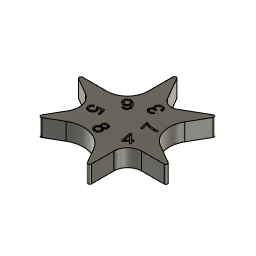
RadiusTool (Autodesk Fusion 360 design; units mm, degrees)
Autodesk Fusion 360 part; units mm, degrees
sketch "Sketch1" plane through (0, 0, 0) normal (0, 0, 1) x (1, 0, 0)
  circle A0 centre (0, 0) radius 20
  line L0 (-4.0272, 3.9759) -> (-4.0272, 20)
  line L1 (-20, 3.9759) -> (-4.0272, 3.9759)
  line L2 (20, -6) -> (6, -6)
  line L3 (6, -6) -> (6, -20)
  dimension "d1" = 40
  constraint coincident A0.centre origin
  constraint horizontal L2
  constraint vertical L3
  constraint horizontal L1
  constraint vertical L0
  measures "d1" diameter of A0
extrude "Extrude1" add sketch "Sketch1" along normal blind 5 contours A0 L0 L1 L2 L3 makes body 1
sketch "Sketch2" plane through (0, 0, 5) normal (0, 0, 1) x (-1, 0, 0)
  arc A0 (-19.0788, 6) -> (4.0272, -19.5904) centre (0, 0) ccw
  line L0 (4.0272, -19.5904) -> (4.0272, -3.9759)
  line L1 (4.0272, -3.9759) -> (19.6008, -3.9759)
  arc A1 (19.6008, -3.9759) -> (-6, 19.0788) centre (0, 0) ccw
  line L2 (-6, 19.0788) -> (-6, 6)
  line L3 (-6, 6) -> (-19.0788, 6)
copy_body "Body->Comp1" bodies 1 removing the originals makes body 2 in component "Component"
move_body "Move1" bodies 2 to x (0.5, -0.866025, 0) y (0.866025, 0.5, 0) z (0, 0, 1) at (0, 0, 0) in component "Component"
sketch "Sketch5" plane through (0, 0, 0) normal (1, 0, 0) x (0, 1, 0)
extrude "Extrude4" cut sketch "Sketch1" along normal blind 5 contours A0 L0 L1 | A0 L2 L3 sketch seen with x (0.5, 0.866025, 0) y (-0.866025, 0.5, 0) z (0, 0, 1) at (0, 0, 0) bodies 2 in component "Component"
extrude "Extrude5" cut sketch "Sketch1" along normal blind 5 contours A0 L0 L1 | A0 L2 L3 sketch seen with x (-1, 0, 0) y (0, -1, 0) z (0, 0, 1) at (0, 0, 0) bodies 2 in component "Component"
fillet "Fillet8" radius 3 1 edges at (-2.1962, -8.1962, 2.5) on bodies 2 in component "Component"
fillet "Fillet9" radius 4 1 edges at (-6, 6, 2.5) on bodies 2 in component "Component"
fillet "Fillet10" radius 5 1 edges at (8.1962, 2.1962, 2.5) on bodies 2 in component "Component"
fillet "Fillet11" radius 6 1 edges at (4.0272, -3.9759, 2.5) on bodies 2 in component "Component"
fillet "Fillet12" radius 7 1 edges at (-5.4568, -1.4997, 2.5) on bodies 2 in component "Component"
fillet "Fillet13" radius 8 1 edges at (1.4297, 5.4756, 2.5) on bodies 2 in component "Component"
fillet "Fillet14" radius 0.5 6 edges at (-6, 18.3442, 2.5) (-18.4467, 6, 2.5) (-12.8865, -14.3682, 2.5) (14.4195, 12.9753, 2.5) (18.8865, -3.9759, 2.5) (4.0272, -18.9753, 2.5) on bodies 2 in component "Component"
sketch "Sketch7" plane through (0, 0, 5) normal (0, 0, 1) x (-1, 0, 0)
  arc A0 (3.0942, -17.3593) -> (4.0272, -17.1093) centre (3.5272, -17.1093) ccw
  line L0 (4.0272, -17.1093) -> (4.0272, -9.9759)
  arc A1 (10.0272, -3.9759) -> (4.0272, -9.9759) centre (10.0272, -9.9759) ccw
  line L1 (10.0272, -3.9759) -> (17.0205, -3.9759)
  arc A2 (17.0205, -3.9759) -> (17.2705, -3.0429) centre (17.0205, -3.4759) ccw
  line L2 (17.2705, -3.0429) -> (12.5263, -0.3038)
  arc A3 (10.6962, 6.5263) -> (12.5263, -0.3038) centre (15.0263, 4.0263) ccw
  line L3 (10.6962, 6.5263) -> (13.4865, 11.3593)
  arc A4 (13.4865, 11.3593) -> (12.8035, 12.0423) centre (13.0535, 11.6093) ccw
  line L4 (12.8035, 12.0423) -> (8.3579, 9.4756)
  arc A5 (-2.5703, 12.4038) -> (8.3579, 9.4756) centre (4.3579, 16.4038) ccw
  line L5 (-2.5703, 12.4038) -> (-5.067, 16.7281)
  arc A6 (-5.067, 16.7281) -> (-6, 16.4781) centre (-5.5, 16.4781) ccw
  line L6 (-6, 16.4781) -> (-6, 10)
  arc A7 (-10, 6) -> (-6, 10) centre (-10, 10) ccw
  line L7 (-10, 6) -> (-16.5806, 6)
  arc A8 (-16.5806, 6) -> (-16.8306, 5.067) centre (-16.5806, 5.5) ccw
  line L8 (-16.8306, 5.067) -> (-11.519, 2.0003)
  arc A9 (-8.9568, -7.5619) -> (-11.519, 2.0003) centre (-15.019, -4.0619) ccw
  line L9 (-8.9568, -7.5619) -> (-11.9535, -12.7522)
  arc A10 (-11.9535, -12.7522) -> (-11.2705, -13.4352) centre (-11.5205, -13.0022) ccw
  line L10 (-11.2705, -13.4352) -> (-4.7942, -9.6962)
  arc A11 (-0.6962, -10.7942) -> (-4.7942, -9.6962) centre (-3.2942, -12.2942) ccw
  line L11 (-0.6962, -10.7942) -> (3.0942, -17.3593)
  line L12 (-3.2168, -7.9766) -> (-0.9529, -8.5832) construction
  line L13 (-0.9529, -8.5832) -> (0.3412, -3.7536) construction
  line L14 (0.3412, -3.7536) -> (-1.9227, -3.147) construction
  line L15 (-1.9227, -3.147) -> (-3.2168, -7.9766) construction
  line L16 (-5.3159, 6.9981) -> (-7.0664, 5.2476) construction
  line L17 (-7.0664, 5.2476) -> (-3.5309, 1.7121) construction
  line L18 (-3.5309, 1.7121) -> (-1.7804, 3.4626) construction
  line L19 (-1.7804, 3.4626) -> (-5.3159, 6.9981) construction
  line L20 (9.243, 1.5792) -> (8.6288, 3.8714) construction
  line L21 (8.6288, 3.8714) -> (3.7992, 2.5773) construction
  line L22 (3.7992, 2.5773) -> (4.4134, 0.2851) construction
  line L23 (4.4134, 0.2851) -> (9.243, 1.5792) construction
  line L24 (4.2315, -5.8439) -> (5.9026, -4.1728) construction
  line L25 (5.9026, -4.1728) -> (2.3671, -0.6372) construction
  line L26 (2.3671, -0.6372) -> (0.696, -2.3083) construction
  line L27 (0.696, -2.3083) -> (4.2315, -5.8439) construction
  line L28 (-7.5796, -0.5504) -> (-6.9799, -2.7884) construction
  line L29 (-6.9799, -2.7884) -> (-2.1503, -1.4943) construction
  line L30 (-2.1503, -1.4943) -> (-2.75, 0.7437) construction
  line L31 (-2.75, 0.7437) -> (-7.5796, -0.5504) construction
  line L32 (3.2162, 7.5935) -> (0.8936, 8.0031) construction
  line L33 (0.8936, 8.0031) -> (0.0254, 3.079) construction
  line L34 (0.0254, 3.079) -> (2.3479, 2.6695) construction
  line L35 (2.3479, 2.6695) -> (3.2162, 7.5935) construction
  text T0 "3" font "Arial" height 5 align ink ink in box 0 x 0 at (-3.2168, -7.9766) x (0.965926, -0.258819) y (0.258819, 0.965926) spacing 1 height is em
  text T1 "4" font "Arial" height 5 align ink ink in box 0 x 0 at (-5.3159, 6.9981) x (-0.707107, -0.707107) y (0.707107, -0.707107) spacing 1 height is em
  text T2 "5" font "Arial" height 5 align ink ink in box 0 x 0 at (9.243, 1.5792) x (-0.258819, 0.965926) y (-0.965926, -0.258819) spacing 1 height is em
  text T3 "6" font "Arial" height 5 align ink ink in box 0 x 0 at (4.2315, -5.8439) x (0.707107, 0.707107) y (-0.707107, 0.707107) spacing 1 height is em
  text T4 "7" font "Arial" height 5 align ink ink in box 0 x 0 at (-7.5796, -0.5504) x (0.258819, -0.965926) y (0.965926, 0.258819) spacing 1 height is em
  text T5 "8" font "Arial" height 5 align ink ink in box 0 x 0 at (3.2162, 7.5935) x (-0.984808, 0.173648) y (-0.173648, -0.984808) spacing 1 height is em
  constraint perpendicular L12 L13
  constraint parallel L12 L14
  constraint parallel L13 L15
  constraint perpendicular L16 L17
  constraint parallel L16 L18
  constraint parallel L17 L19
  constraint perpendicular L20 L21
  constraint parallel L20 L22
  constraint parallel L21 L23
  constraint perpendicular L24 L25
  constraint parallel L24 L26
  constraint parallel L25 L27
  constraint perpendicular L28 L29
  constraint parallel L28 L30
  constraint parallel L29 L31
  constraint perpendicular L32 L33
  constraint parallel L32 L34
  constraint parallel L33 L35
extrude "Extrude6" cut sketch "Sketch7" against normal blind 0.5 text T0 T4 T1 T5 T2 T3 sketch seen with x (-1, 0, 0) y (0, -1, 0) z (0, 0, 1) at (0, 0, 0) bodies 2 in component "Component"
component "Component" placed x (-1, 0, 0) y (0, -1, 0) z (0, 0, 1) at (0, 0, 0)
